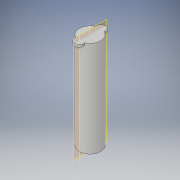
# Autodesk Inventor part: reducedLargeSyrginePlunger
Saved by Autodesk Inventor 2018 (Build 220112000, 112)
## iProperties
Created: 2020-03-29
Part Number: reducedLargeSyrginePlunger
Material: Generic
Document SubType Name: Modeling
Designer: Jesse R-B
Density: 1 g/cm^3
Appearance: Default
Author: Jesse R-B
Autodesk Inventor part; units mm, degrees
ref_plane "XZ Plane" through (0, 0, 0) normal (0, 1, 0) x (-1, 0, 0)
ref_plane "XY Plane" through (0, 0, 0) normal (0, 0, 1) x (1, 0, 0)
sketch "Sketch1" plane through (0, 0, 0) normal (0, 1, 0) x (-1, 0, 0)
  circle A0 centre (0, 0) radius 22.86
  dimension "d0" = 45.72
  constraints: 1 centre point, 1 coincident
  measures "d0" diameter of A0
extrude "Extrusion1" add sketch "Sketch1" along normal blind 200.66
sketch "Sketch2" plane through (0, 200.66, 0) normal (0, 1, 0) x (1, 0, 0)
  circle A0 centre (0, 0) radius 22.86 projected
  circle A1 centre (0, -22.86) radius 9.906
  circle A2 centre (0, 22.86) radius 9.906
  dimension "d3" = 19.812
  dimension "d4" = 19.812
  constraints: 2 centre point, 2 point on circle
  measures "d3" diameter of A1
  measures "d4" diameter of A2
extrude "Extrusion2" add sketch "Sketch2" along normal blind 5.08
ref_plane "Work Plane1" through (22.86, 0, 0) normal (1, 0, 0) x (0, 1, 0)
body "Solid1"
